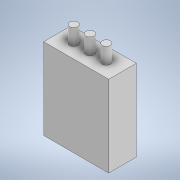
# Autodesk Inventor part: Hall Sensor
Saved by Autodesk Inventor 2021 (Build 250183000, 183)
## iProperties
Created: 2021-08-31
Part Number: Hall Sensor
Material: Genérico
Document SubType Name: Modeling
Designer: Diego.labarca
Density: 1 g/cm^3
Appearance: Valor por defecto
Author: Diego.labarca
Autodesk Inventor part; units mm, degrees
ref_plane "YZ Plane" through (0, 0, 0) normal (1, 0, 0) x (0, 1, 0)
ref_plane "XZ Plane" through (0, 0, 0) normal (0, 1, 0) x (-1, 0, 0)
ref_plane "XY Plane" through (0, 0, 0) normal (0, 0, 1) x (1, 0, 0)
sketch "Boceto1" plane through (0, 0, 0) normal (0, 0, 1) x (1, 0, 0)
  line L0 (-2, 2.5) -> (2, 2.5)
  line L1 (2, 2.5) -> (2, -2.5)
  line L2 (2, -2.5) -> (-2, -2.5)
  line L3 (-2, -2.5) -> (-2, 2.5)
  line L4 (0, -3.5) -> (0, 3.5) projected
  line L5 (-2.8, 0) -> (2.8, 0) projected
  point P0 (0, 0)
  dimension "d0" = 4
  dimension "d1" = 5
  constraints: 8 end point, 2 parallel, 1 horizontal, 1 perpendicular, 2 other
  measures "d0" distance of L1.end L2.end
  measures "d1" distance of L0.end L1.end
extrude "Extrusión1" add sketch "Boceto1" along normal blind 1.7
sketch "Boceto2" plane through (-2, 2.5, 0) normal (0, 1, 0) x (1, 0, 0)
  circle A0 centre (1, -0.85) radius 0.25
  circle A1 centre (2, -0.85) radius 0.25
  circle A2 centre (3, -0.85) radius 0.25
  line L0 (4, 0) -> (4, -1.7) projected
  line L1 (0, 0) -> (0, -1.7) projected
  line L2 (4, -1.7) -> (0, -1.7) projected
  point P0 (2, 0)
  dimension "d4" = 0.5
  dimension "d5" = 0.5
  dimension "d6" = 0.5
  dimension "d8" = 1
  dimension "d9" = 1
  dimension "d10" = 4
  dimension "d11" = 2
  dimension "d12" = 0.85
  dimension "d13" = 1.7
  dimension "d14" = 0.85
  dimension "d15" = 0.85
  constraints: 3 centre point
  measures "d4" diameter of A0
  measures "d5" diameter of A1
  measures "d6" diameter of A2
  measures "d8" distance of A1.centre A0.centre
  measures "d9" distance of A2.centre A1.centre
  measures "d10" distance between parallel lines of L0 L1
  measures "d11" distance from line of L1 A1.centre
  measures "d12" distance from line of L2 A1.centre
  measures "d13" distance of L0.start L0.end
  measures "d14" distance from line of L2 A0.centre
  measures "d15" distance from line of L2 A2.centre
extrude "Extrusión2" add sketch "Boceto2" along normal blind 1
equation "\"d9\" = d8"
equation "\"d11\" = 0.5 * d10"
equation "\"d12\" = 0.5 * d13"
equation "\"d14\" = d12"
equation "\"d15\" = d12"
